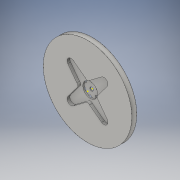
# Autodesk Inventor part: Aidan Sherry Wheel
Saved by Autodesk Inventor 2016 (Build 200138000, 138)
## iProperties
Created: 2016-10-14
Part Number: Aidan Sherry Wheel
Material: Generic
Document SubType Name: Modeling
Designer: sherra
Density: 1 g/cm^3
Appearance: Default
Author: sherra
Autodesk Inventor part; units mm, degrees
ref_plane "YZ Plane" through (0, 0, 0) normal (1, 0, 0) x (0, 1, 0)
ref_plane "XZ Plane" through (0, 0, 0) normal (0, 1, 0) x (-1, 0, 0)
ref_plane "XY Plane" through (0, 0, 0) normal (0, 0, 1) x (1, 0, 0)
sketch "Sketch1" plane through (0, 0, 0) normal (0, 0, 1) x (1, 0, 0)
  circle A0 centre (0, 0) radius 31.5468
  dimension "d0" = 63.0936
  constraints: 1 centre point, 1 coincident
  measures "d0" diameter of A0
extrude "Extrusion1" add sketch "Sketch1" along normal blind 3.556
sketch "Sketch5" plane through (0, 0, 3.556) normal (0, 0, 1) x (1, 0, 0)
  arc A0 (1.5256, -7.6067) -> (-1.5256, -7.6067) centre (0, -8.5367) ccw
  line L0 (1.5256, -7.6067) -> (10.0877, -14.0155)
  arc A1 (10.0877, -14.0155) -> (14.0155, -10.0877) centre (11.7691, -11.7691) ccw
  line L1 (14.0155, -10.0877) -> (7.6067, -1.5256)
  arc A2 (7.6067, 1.5256) -> (7.6067, -1.5256) centre (8.5367, 0) ccw
  line L2 (7.6067, 1.5256) -> (14.0155, 10.0877)
  arc A3 (14.0155, 10.0877) -> (10.0877, 14.0155) centre (11.7691, 11.7691) ccw
  line L3 (10.0877, 14.0155) -> (1.5256, 7.6067)
  arc A4 (-1.5256, 7.6067) -> (1.5256, 7.6067) centre (0, 8.5367) ccw
  line L4 (-1.5256, 7.6067) -> (-10.0877, 14.0155)
  arc A5 (-10.0877, 14.0155) -> (-14.0155, 10.0877) centre (-11.7691, 11.7691) ccw
  line L5 (-14.0155, 10.0877) -> (-7.6067, 1.5256)
  arc A6 (-7.6067, -1.5256) -> (-7.6067, 1.5256) centre (-8.5367, 0) ccw
  line L6 (-7.6067, -1.5256) -> (-14.0155, -10.0877)
  arc A7 (-14.0155, -10.0877) -> (-10.0877, -14.0155) centre (-11.7691, -11.7691) ccw
  line L7 (-10.0877, -14.0155) -> (-1.5256, -7.6067)
  circle A8 centre (12.339, -12.339) radius 0.75
  circle A9 centre (9.8641, -9.8641) radius 0.75
  circle A10 centre (7.3893, -7.3893) radius 0.75
  circle A11 centre (4.9144, -4.9144) radius 0.75
  circle A12 centre (12.339, 12.339) radius 0.75
  circle A13 centre (9.8641, 9.8641) radius 0.75
  circle A14 centre (7.3893, 7.3893) radius 0.75
  circle A15 centre (4.9144, 4.9144) radius 0.75
  circle A16 centre (-12.339, 12.339) radius 0.75
  circle A17 centre (-9.8641, 9.8641) radius 0.75
  circle A18 centre (-7.3893, 7.3893) radius 0.75
  circle A19 centre (-4.9144, 4.9144) radius 0.75
  circle A20 centre (-12.339, -12.339) radius 0.75
  circle A21 centre (-9.8641, -9.8641) radius 0.75
  circle A22 centre (-7.3893, -7.3893) radius 0.75
  circle A23 centre (-4.9144, -4.9144) radius 0.75
  circle A24 centre (0, 0) radius 3.6
  constraints: 25 centre point, 16 end point, 16 point on circle
extrude "Extrusion4" cut sketch "Sketch5" against normal blind 1.9558 contours A0 L7 A7 L6 A6 L5 A5 L4 A4 L3 A3 L2 A2 L1 A1 L0 | A8 | A9 | A10 | A11 | A12 | A13 | A14 | A15 | A16 | A17 | A18 | A19 | A20 | A21 | A22 | A23 | A24
sketch "Sketch6" plane through (0, 0, 0) normal (0, 1, 0) x (-1, 0, 0)
  point P0 (0, 0)
sketch "Sketch7" plane through (0, 0, 0) normal (0, 1, 0) x (-1, 0, 0)
  point P0 (0, 0)
sketch "Sketch8" plane through (0, 0, 0) normal (1, 0, 0) x (0, 1, 0)
  line L0 (31.5468, 0) -> (31.5468, 3.556) projected
  circle A0 centre (31.5468, 1.778) radius 1.7361
  line L1 (0, 0) -> (0, 3.556)
  line L2 (31.5468, 3.556) -> (-31.5468, 3.556) projected
  constraints: 2 end point, 2 midpoint, 1 centre point
revolve "Revolution1" cut sketch "Sketch8" angle 360 about axis through (0, 0, 0) along (0, 0, 1)
sketch "Sketch9" plane through (0, 0, 1.6002) normal (0, 0, 1) x (1, 0, 0)
  circle A0 centre (0, 0) radius 1.27
  circle A1 centre (0, 0) radius 5.2705
  constraints: 2 centre point, 2 coincident
extrude "Extrusion5" cut sketch "Sketch9" along normal mid plane 25.4 contours A0
sketch "Sketch10" plane through (0, 0, 3.556) normal (0, 0, 1) x (1, 0, 0)
  point P0 (0, 0)
sketch "Sketch11" plane through (0, 0, 1.6002) normal (0, 0, 1) x (1, 0, 0)
  circle A0 centre (0, 0) radius 5.2705
  constraints: 1 centre point, 1 coincident
extrude "Extrusion6" cut sketch "Sketch11" against normal blind 1.016
sketch "Sketch13" plane through (0, 0, 0) normal (0, 0, -1) x (-1, 0, 0)
  circle A0 centre (0, 0) radius 29.8107 projected
  line L0 (23.7905, 8.4223) -> (19.1073, 10.3576)
  line L1 (19.1073, 10.3576) -> (19.1073, 17.0437)
  line L2 (19.1073, 17.0437) -> (23.7905, 15.1084)
  line L3 (23.7905, 15.1084) -> (23.7905, 8.4223)
  line L4 (16.7989, 19.0048) -> (14.678, 20.9264)
  line L5 (14.678, 20.9264) -> (12.4752, 19.1187)
  line L6 (12.4752, 19.1187) -> (12.4752, 9.951)
  line L7 (16.7989, 19.0048) -> (16.7989, 9.39)
  line L8 (29.8101, -0.1885) -> (-29.8107, 0) construction
  line L9 (29.8101, -0.1885) -> (-29.8107, 0) construction
  line L10 (4.1485, 5.1436) -> (12.4752, 9.951)
  line L11 (6.2117, 1.3422) -> (14.1511, 5.926)
  line L12 (3.5448, 2.346) -> (6.2117, 1.3422)
  line L13 (4.1485, 5.1436) -> (3.5448, 2.346)
  line L14 (22.4779, 1.1186) -> (14.1511, 5.926)
  line L15 (24.7384, 4.8061) -> (16.7989, 9.39)
  line L16 (25.2024, 1.9946) -> (24.7384, 4.8061)
  line L17 (22.4779, 1.1186) -> (25.2024, 1.9946)
  line L18 (-22.9413, 8.4223) -> (-18.2582, 10.3576)
  line L19 (-18.2582, 10.3576) -> (-18.2582, 17.0437)
  line L20 (-18.2582, 17.0437) -> (-22.9413, 15.1084)
  line L21 (-22.9413, 15.1084) -> (-22.9413, 8.4223)
  line L22 (-18.3239, -10.4304) -> (-18.3662, -17.1164)
  line L23 (-18.3662, -17.1164) -> (-23.037, -15.1516)
  line L24 (-23.037, -15.1516) -> (-22.9947, -8.4656)
  line L25 (-22.9947, -8.4656) -> (-18.3239, -10.4304)
  line L26 (19.1731, -10.4304) -> (19.2154, -17.1164)
  line L27 (23.8439, -8.4656) -> (19.1731, -10.4304)
  line L28 (23.8862, -15.1516) -> (23.8439, -8.4656)
  line L29 (19.2154, -17.1164) -> (23.8862, -15.1516)
  line L30 (5.0802, 24.7659) -> (0.4246, 27.6234)
  line L31 (-4.2403, 24.7659) -> (0.4246, 21.9027)
  line L32 (5.0802, 24.7659) -> (0.4246, 21.9027)
  line L33 (0.4246, 27.6234) -> (-4.2403, 24.7659)
  line L34 (4.9229, -24.9861) -> (0.2493, -27.8141)
  line L35 (-4.3975, -24.9271) -> (0.2855, -22.0935)
  line L36 (4.9229, -24.9861) -> (0.2855, -22.0935)
  line L37 (0.2493, -27.8141) -> (-4.3975, -24.9271)
  line L38 (-10.6543, 22.7592) -> (-10.1902, 19.9477)
  line L39 (-7.9297, 23.6352) -> (-10.6543, 22.7592)
  line L40 (-10.1902, 19.9477) -> (-2.2508, 15.3638)
  line L41 (-7.9297, 23.6352) -> (0.397, 18.8278)
  line L42 (-2.2508, 5.749) -> (-0.1298, 3.8274)
  line L43 (-0.1298, 3.8274) -> (2.073, 5.6351)
  line L44 (15.1978, 25.3066) -> (-14.7759, -26.2323) construction
  line L45 (15.1978, 25.3066) -> (-14.7759, -26.2323) construction
  line L46 (-2.2508, 5.749) -> (-2.2508, 15.3638)
  line L47 (2.073, 5.6351) -> (2.073, 14.8028)
  line L48 (10.3997, 19.6102) -> (2.073, 14.8028)
  line L49 (10.3997, 19.6102) -> (11.0033, 22.4078)
  line L50 (8.3364, 23.4116) -> (0.397, 18.8278)
  line L51 (11.0033, 22.4078) -> (8.3364, 23.4116)
  line L52 (-24.9077, 1.7372) -> (-22.2408, 0.7333)
  line L53 (-24.304, 4.5348) -> (-24.9077, 1.7372)
  line L54 (-22.2408, 0.7333) -> (-14.3014, 5.3172)
  line L55 (-24.304, 4.5348) -> (-15.9773, 9.3422)
  line L56 (-5.9746, 0.5098) -> (-3.2501, 1.3858)
  line L57 (-3.2501, 1.3858) -> (-3.7142, 4.1973)
  line L58 (-14.1877, 25.3995) -> (15.4594, -26.328) construction
  line L59 (-14.1877, 25.3995) -> (15.4594, -26.328) construction
  line L60 (-5.9746, 0.5098) -> (-14.3014, 5.3172)
  line L61 (-3.7142, 4.1973) -> (-11.6536, 8.7811)
  line L62 (-11.6536, 18.396) -> (-11.6536, 8.7811)
  line L63 (-11.6536, 18.396) -> (-13.7745, 20.3175)
  line L64 (-15.9773, 18.5099) -> (-15.9773, 9.3422)
  line L65 (-13.7745, 20.3175) -> (-15.9773, 18.5099)
  line L66 (-13.8288, -21.1176) -> (-11.626, -19.3099)
  line L67 (-15.9498, -19.196) -> (-13.8288, -21.1176)
  line L68 (-11.626, -19.3099) -> (-11.626, -10.1423)
  line L69 (-15.9498, -19.196) -> (-15.9498, -9.5812)
  line L70 (-3.2993, -5.3348) -> (-2.6957, -2.5372)
  line L71 (-2.6957, -2.5372) -> (-5.3626, -1.5334)
  line L72 (-28.961, -0.0027) -> (30.6599, -0.1912) construction
  line L73 (-28.961, -0.0027) -> (30.6599, -0.1912) construction
  line L74 (-3.2993, -5.3348) -> (-11.626, -10.1423)
  line L75 (-5.3626, -1.5334) -> (-13.302, -6.1172)
  line L76 (-21.6287, -1.3098) -> (-13.302, -6.1172)
  line L77 (-21.6287, -1.3098) -> (-24.3533, -2.1858)
  line L78 (-23.8892, -4.9974) -> (-15.9498, -9.5812)
  line L79 (-24.3533, -2.1858) -> (-23.8892, -4.9974)
  line L80 (11.5035, -22.9504) -> (11.0394, -20.1389)
  line L81 (8.7789, -23.8264) -> (11.5035, -22.9504)
  line L82 (11.0394, -20.1389) -> (3.0999, -15.555)
  line L83 (8.7789, -23.8264) -> (0.4522, -19.019)
  line L84 (3.0999, -5.9402) -> (0.979, -4.0186)
  line L85 (0.979, -4.0186) -> (-1.2238, -5.8263)
  line L86 (-14.3487, -25.4978) -> (15.625, 26.0411) construction
  line L87 (-14.3487, -25.4978) -> (15.625, 26.0411) construction
  line L88 (3.0999, -5.9402) -> (3.0999, -15.555)
  line L89 (-1.2238, -5.8263) -> (-1.2238, -14.994)
  line L90 (-9.5505, -19.8014) -> (-1.2238, -14.994)
  line L91 (-9.5505, -19.8014) -> (-10.1542, -22.599)
  line L92 (-7.4873, -23.6028) -> (0.4522, -19.019)
  line L93 (-10.1542, -22.599) -> (-7.4873, -23.6028)
  line L94 (25.7568, -1.9284) -> (23.09, -0.9246)
  line L95 (25.1532, -4.726) -> (25.7568, -1.9284)
  line L96 (23.09, -0.9246) -> (15.1505, -5.5084)
  line L97 (25.1532, -4.726) -> (16.8265, -9.5334)
  line L98 (6.8238, -0.701) -> (4.0992, -1.577)
  line L99 (4.0992, -1.577) -> (4.5633, -4.3885)
  line L100 (15.0369, -25.5907) -> (-14.6103, 26.1367) construction
  line L101 (15.0369, -25.5907) -> (-14.6103, 26.1367) construction
  line L102 (6.8238, -0.701) -> (15.1505, -5.5084)
  line L103 (4.5633, -4.3885) -> (12.5027, -8.9723)
  line L104 (12.5027, -18.5872) -> (12.5027, -8.9723)
  line L105 (12.5027, -18.5872) -> (14.6237, -20.5087)
  line L106 (16.8265, -18.7011) -> (16.8265, -9.5334)
  line L107 (14.6237, -20.5087) -> (16.8265, -18.7011)
  point P0 (14.4751, 8.4223)
  point P1 (14.4751, -8.932)
  point P2 (0.4246, -0.0956)
  point P3 (0.0731, 16.3314)
  point P4 (0.4246, -0.0956)
  point P5 (-13.9774, 7.8135)
  point P6 (0.4246, -0.0956)
  point P7 (-13.6259, -8.6136)
  point P8 (0.4246, -0.0956)
  point P9 (0.7761, -16.5227)
  point P10 (0.4246, -0.0956)
  point P11 (14.8266, -8.0047)
  constraints: 216 end point, 8 symmetric about line, 6 point on line, 3 parallel, 3 vertical, 2 point on circle, 1 collinear
extrude "Extrusion7" cut sketch "Sketch13" against normal blind 0.762 contours L0 L1 L2 L3 | L7 L15 L16 L17 L14 L11 L12 L13 L10 L6 L5 L4 | L21 L20 L19 L18 | L22 L23 L24 L25 | L27 L28 L29 L26 | L32 L31 L33 L30 | L34 L37 L35 L36 | L39 L41 L50 L51 L49 L48 L47 L43 L42 L46 L40 L38 | L53 L55 L64 L65 L63 L62 L61 L57 L56 L60 L54 L52 | L67 L69 L78 L79 L77 L76 L75 L71 L70 L74 L68 L66 | L81 L83 L92 L93 L91 L90 L89 L85 L84 L88 L82 L80 | L95 L97 L106 L107 L105 L104 L103 L99 L98 L102 L96 L94
body "Solid1"
